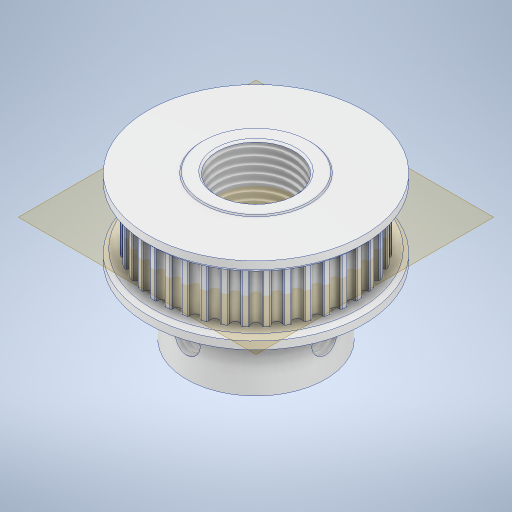
# Autodesk Inventor part: 6mm 40T GT2 Timing Pulley SFU1204 Bore
Saved by Autodesk Inventor 2024 (Build 280153000, 153)
## iProperties
Created: 2023-06-15
Part Number: 6mm 40T GT2 Timing Pulley SFU1204 Bore
Material: Aluminum 6061
Document SubType Name: Modeling
Designer: Ishaan
Density: 2.7 g/cm^3
Appearance: Aluminum - Flat
Author: Ishaan
Autodesk Inventor part; units mm, degrees
ref_plane "XZ Plane" through (0, 0, 0) normal (0, 1, 0) x (-1, 0, 0)
sketch "Sketch1" plane through (0, 0, 0) normal (0, 0, 1) x (1, 0, 0)
  line L0 (0, 0) -> (-9, 0)
  line L1 (-9, 0) -> (-9, 10.2)
  line L2 (-9, 10.2) -> (0, 10.2)
  line L3 (0, 10.2) -> (0, 0)
  line L4 (0, 10.2) -> (-12.48, 10.2)
  line L5 (-12.48, 10.2) -> (-12.48, 17.2)
  line L6 (-12.48, 17.2) -> (0, 17.2)
  line L7 (0, 17.2) -> (0, 10.2)
  line L8 (0, 17.2) -> (-14, 17.2)
  line L9 (-14, 18.7) -> (0, 18.7)
  line L10 (0, 18.7) -> (0, 17.2)
  line L11 (0, 18.7) -> (-5, 18.7)
  line L12 (-5, 18.7) -> (-5, 0)
  line L13 (-5, 0) -> (-0.9661, 0)
  line L14 (-9, 10.2) -> (-14, 10.2)
  line L15 (-14, 10.2) -> (-14, 8.7)
  line L16 (-14, 8.7) -> (-9, 8.7)
  line L17 (-9, 8.7) -> (-9, 10.2)
  line L18 (-14, 18.7) -> (-14, 17.2)
  line L19 (-5, 18.7) -> (-7, 18.7)
  line L20 (-7, 18.7) -> (-7, 18.85)
  line L21 (-7, 18.85) -> (-5, 18.85)
  line L22 (-5, 18.85) -> (-5, 18.7)
  line L23 (-5, 0) -> (-7, 0)
  line L24 (-7, 0) -> (-7, -0.15)
  line L25 (-7, -0.15) -> (-5, -0.15)
  line L26 (-5, -0.15) -> (-5, 0)
  line L27 (-5, -0.15) -> (-4, -0.15)
  line L28 (-4, -0.15) -> (-4, 10.2)
  line L29 (-4, 10.2) -> (-5, 10.2)
  line L30 (-5, 10.2) -> (-5, -0.15)
  point P0 (-12.48, 17.2)
  point P1 (-6.11, 10.1197)
  point P2 (-5, 17.2)
  point P3 (-5, 10.2)
  point P4 (-7, 0)
  dimension "d1" = 5
  dimension "d3" = 7
  dimension "d5" = 12.48
  dimension "d35" = 8.7
  dimension "d36" = 9
  dimension "d38" = 14
  dimension "d39" = 1.5
  dimension "d40" = 2
  dimension "d41" = 0.15
  dimension "d42" = 2
  dimension "d43" = 0.15
  dimension "d44" = 4
  constraints: 62 end point, 14 parallel, 8 horizontal, 7 perpendicular, 3 collinear, 2 point on line, 1 vertical
  measures "d1" distance between parallel lines of L12 L3
  measures "d3" distance between parallel lines of L2 L8
  measures "d5" distance between parallel lines of L7 L5
  measures "d35" distance between parallel lines of L16 L0
  measures "d36" distance from line of L0.start L1
  measures "d38" distance of L9.start L9.end
  measures "d39" distance between parallel lines of L16 L14
  measures "d40" distance of L20.end L21.end
  measures "d41" distance of L19.end L20.end
  measures "d42" distance of L25.end L24.end
  measures "d43" distance of L24.end L23.end
  measures "d44" distance between parallel lines of L3 L28
revolve "Revolution1" add sketch "Sketch1" angle 360 about axis through (0, 17.2, 0) along (0, -1, 0) contours L28 L27 L26 L0 | L0 L12 L2 L28 | L26 L25 L24 L0 | L0 L1 L2 L12 | L2 L4 L5 L6 L12 | L6 L8 L18 L9 L12 | L1 L16 L15 L14 L4 | L9 L20 L21 L22
chamfer "Chamfer3" distance 1 angle 45 1 edges at (4, 10.2, 0)
thread "Thread1" size "M10x1" class "6H" standard "ANSI Metric M Profile" full length
chamfer "Chamfer4" distance 0.25 angle 45 2 edges at (5, 18.85, 0) (4, -0.15, 0)
chamfer "Chamfer2" distance 0.5 angle 45 2 edges at (14, 17.2, 0) (14, 10.2, 0)
chamfer "Chamfer1" distance 0.15 angle 45 2 edges at (7, 18.85, 0) (7, -0.15, 0)
ref_plane "Work Plane2" through (0, 4.35, 0) normal (0, -1, 0) x (1, 0, 0)
sketch "Sketch3" plane through (0, 0, 0) normal (1, 0, 0) x (0, 1, 0)
  line L0 (4.35, -19.6) -> (4.35, 19.6) projected
  line L1 (-0.71, 0) -> (4.26, 0) projected
  point P0 (0, 0)
  point P1 (4.35, 0)
  constraints: 1 midpoint, 1 point on line
hole "Hole1" at (0, 4.35, 0) direction (1, 0, 0) diameter 3.242 end through all thread size "M4x0.7" class "6H" standard "ANSI Metric M Profile"
ref_plane "Work Plane3" through (0, 0, 0) normal (-0.7071, 0, 0.7071) x (0, -1, 0)
mirror "Mirror2" about plane through (0, 0, 0) normal (-0.7071, 0, 0.7071) of "Hole1"
sketch "Sketch5" plane through (0, 17.2, 0) normal (0, -1, 0) x (1, 0, 0)
  circle A0 centre (0, 0) radius 12.48 projected
  circle A1 centre (0, 0) radius 5 projected
  circle A2 centre (0, 0) radius 12.48 construction
  arc A3 (-0.7131, -12.4596) -> (0.7131, -12.4596) centre (0, 0) ccw
  arc A4 (0.5547, -12.3046) -> (0.7131, -12.4596) centre (0.7046, -12.3099) ccw
  arc A5 (-0.7131, -12.4596) -> (-0.5547, -12.3046) centre (-0.7046, -12.3099) ccw
  arc A6 (0.5547, -12.3046) -> (-0.5547, -12.3046) centre (0, -12.285) ccw
  circle A7 centre (0, 0) radius 13.5 projected
  point P0 (0, 0)
  point P1 (-0.7131, -12.4596)
  point P2 (0.7131, -12.4596)
  dimension "d23" = 0.15
  dimension "d24" = 0.555
  dimension "d25" = 0.75
  constraints: 8 point on circle, 6 tangent, 5 centre point, 1 coincident, 1 concentric, 1 equal radius, 1 vertical alignment
  measures "d23" radius of A4
  measures "d24" radius of A6
extrude "Extrusion3" cut sketch "Sketch5" along normal up to surface (7 mm away) contours A5 A6 A4 A0 picked at (-0.0228, -12.2299)
pattern_circular "Circular Pattern1" count 40 over 360 about axis through (0, 14.525, 0) along (0, -1, 0) of "Extrusion3"
chamfer "Chamfer5" distance 0.25 angle 45 1 edges at (9, 8.7, 0)
ref_plane "Work Plane4" through (0, 13.7, 0) normal (0, 1, 0) x (1, 0, 0)
body "Solid1"
